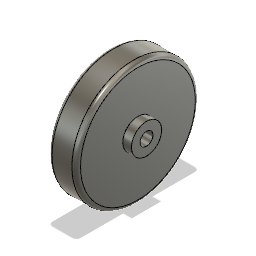
wheel v1 (Autodesk Fusion 360 design; units mm, degrees)
Autodesk Fusion 360 part; units mm, degrees
sketch "スケッチ1" plane through (0, 0, 0) normal (1, 0, 0) x (0, 0, -1)
  circle A0 centre (0, 0) radius 14.3
  dimension "d1" = 28.6
  measures "d1" diameter of A0
extrude "押し出し1" add sketch "スケッチ1" along normal blind 6.6
sketch "スケッチ2" plane through (6.6, 0, 0) normal (1, 0, 0) x (0, 0, -1)
  circle A0 centre (0, 0) radius 14.3
  circle A1 centre (0, 0) radius 3.5
  dimension "d4" = 7
  measures "d4" diameter of A1
extrude "押し出し2" add sketch "スケッチ2" along normal blind 2 contours A1
sketch "スケッチ3" plane through (8.6, 0, 0) normal (1, 0, 0) x (0, 0, -1)
  circle A0 centre (0, 0) radius 3.5
  circle A1 centre (0, 0) radius 1.5
  dimension "d7" = 3
  measures "d7" diameter of A1
extrude "押し出し3" cut sketch "スケッチ3" along normal mid plane 17.6 contours A1
fillet "フィレット1" radius 1 1 edges at (0, -5.1711, 13.3323)
fillet "フィレット2" radius 1 1 edges at (6.6, -5.1711, 13.3323)
